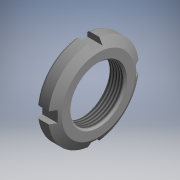
# Autodesk Inventor part: KM 4
Saved by Autodesk Inventor 2017.3 (Build 213256000, 256)
## iProperties
Part Number: KM 4
Material: Generic
Catalog Web Link: www.cadenas.de
Description: ANL_001-KM(L) and HM .. T lock nuts
Vendor: SKF
Document SubType Name: Modeling
Designer: partserver
Manufacturer: SKF
Mass: 25 g
Surface Area: 18.2354 cm^2
Volume: 2.6965 cm^3
Density: 1 g/cm^3
Appearance: PSOLRGB-175-175-175
Category: PARTsolutions
Company: SKF
Title: KM 4
Author: Cadenas PARTsolutions
Comments: KM(L) and HM .. T lock nuts
PSOL_IDENT_0: {$CADENAS_DATA\23d-libs\skf\bearings_units_and_housings\bearing_accessories\lock_nuts\anl_001.prj},1
PSOL_IDENT_1: 51 {VTYP=3D},{NB=KM 4},{LINA=KM 4},{NN=ANL_001},{DATE=23.12.2020 11:57:30},{GEOMDATE=27.11.2020 10:1
PSOL_IDENT_2: 1:00},{VERSION=},{LINEID=3230},{WBVAR=},{WBNUMERIC=}  {NB=KM 4},{LINA=KM 4},{KT=DUMMY},{DESIGNATION=
PSOL_IDENT_3: KM 4},{G=M 20x1},{DD=20.000},{TP=1.000},{DD3=32.000},{B=6.000},{DD1=26.000},{DD2=MIN},{B3=MIN},{B5=M
PSOL_IDENT_4: IN},{BB=4.000},{HH=2.000},{MASS=0.025},{SD=HN 4},{WD=MB 4},{DESIGN=locknut_km},{LNB=34.000},{POPULAR=
PSOL_IDENT_5: Yes},{EB=},{LOAD=24},{WDX=MB 4},{KH=}
NB: KM 4
NN: ANL_001
NT: KM(L) and HM .. T lock nuts
NBSYN: $DESIGNATION.
LINA: KM 4
CATALOG: SKF
DESIGNATION: KM 4
G: M 20x1
DD: 20
DD3: 32
B: 6
WD: MB 4
POPULAR: Yes
LOAD: 24
WDX: MB 4
SUPPLIER: SKF
ARTICLENO: KM 4
BOMINFO: KM 4
CREATOR: CADENAS GmbH
Autodesk Inventor part; units mm, degrees
sketch "Sketch_3" plane through (0, 0, 0) normal (0, 0, 1) x (1, 0, 0)
  line L0 (68, 0) -> (-68, 0)
  line L1 (0, 10) -> (0.5415, 9.4585)
  line L2 (0.5415, 9.4585) -> (5.4585, 9.4585)
  line L3 (5.4585, 9.4585) -> (6, 10)
  line L4 (6, 10) -> (6, 15)
  arc A0 (6, 15) -> (5, 16) centre (5, 15) ccw
  line L5 (5, 16) -> (1.7321, 16)
  line L6 (1.7321, 16) -> (0, 13)
  line L7 (0, 13) -> (0, 10)
  constraints: 16 end point, 2 point on circle, 1 centre point
revolve "Revolution1" add sketch "Sketch_3" angle 360 about axis through (68, 0, 0) along (-1, 0, 0)
thread "Thread1" size "M20x1" class "6H" standard "ISO Metric profile" full length
sketch "Sketch_6" plane through (0, 0, 0) normal (1, 0, 0) x (0, 1, 0)
  circle A0 centre (0, 0) radius 32
  line L0 (2, 20.9045) -> (2, 13.8745)
  line L1 (2, 13.8745) -> (-2, 13.8745)
  line L2 (-2, 13.8745) -> (-2, 20.9045)
  arc A1 (-2, 20.9045) -> (-20.9045, 2) centre (0, 0) ccw
  line L3 (-20.9045, 2) -> (-13.8745, 2)
  line L4 (-13.8745, 2) -> (-13.8745, -2)
  line L5 (-13.8745, -2) -> (-20.9045, -2)
  arc A2 (-20.9045, -2) -> (-2, -20.9045) centre (0, 0) ccw
  line L6 (-2, -20.9045) -> (-2, -13.8745)
  line L7 (-2, -13.8745) -> (2, -13.8745)
  line L8 (2, -13.8745) -> (2, -20.9045)
  arc A3 (2, -20.9045) -> (20.9045, -2) centre (0, 0) ccw
  line L9 (20.9045, -2) -> (13.8745, -2)
  line L10 (13.8745, -2) -> (13.8745, 2)
  line L11 (13.8745, 2) -> (20.9045, 2)
  arc A4 (20.9045, 2) -> (2, 20.9045) centre (0, 0) ccw
  constraints: 24 end point, 8 point on circle, 5 centre point
extrude "Extrusion1" cut sketch "Sketch_6" along normal blind 12
ref_plane "km_XY" through (6, 0, 0) normal (1, 0, 0) x (0, 0, -1)
ref_plane "km_YZ" through (6, 0, 0) normal (0, 0, -1) x (0, 1, 0)
ref_plane "km_ZX" through (6, 0, 0) normal (0, 1, 0) x (1, 0, 0)
ref_plane "km2_XY" through (6, 0, 0) normal (1, 0, 0) x (0, 0, -1)
ref_plane "km2_YZ" through (6, 0, 0) normal (0, 0, -1) x (0, 1, 0)
ref_plane "km2_ZX" through (6, 0, 0) normal (0, 1, 0) x (1, 0, 0)
ref_plane "ln_XY" through (0, 0, 0) normal (0, 1, 0) x (1, 0, 0)
ref_plane "ln_YZ" through (0, 0, 0) normal (1, 0, 0) x (0, 0, -1)
ref_plane "ln_ZX" through (0, 0, 0) normal (0, 0, -1) x (0, 1, 0)
ref_plane "nut_XY" through (0, 0, 0) normal (1, 0, 0) x (0, 0, -1)
ref_plane "nut_YZ" through (0, 0, 0) normal (0, 0, -1) x (0, 1, 0)
ref_plane "nut_ZX" through (0, 0, 0) normal (0, 1, 0) x (1, 0, 0)
body "Solid1"
